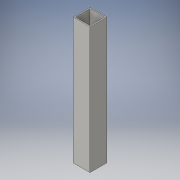
# Autodesk Inventor part: gripper arm bracket
Saved by Autodesk Inventor 2016 SP2 (Build 200236200, 236)
## iProperties
Created: 2018-02-13
Part Number: gripper arm bracket
Material: Generic
Document SubType Name: Modeling
Designer: CAD
Density: 1 g/cm^3
Appearance: Default
Author: CAD
Autodesk Inventor part; units mm, degrees
ref_plane "YZ Plane" through (0, 0, 0) normal (1, 0, 0) x (0, 1, 0)
ref_plane "XZ Plane" through (0, 0, 0) normal (0, 1, 0) x (-1, 0, 0)
ref_plane "XY Plane" through (0, 0, 0) normal (0, 0, 1) x (1, 0, 0)
sketch "Sketch1" plane through (0, 0, 0) normal (0, 1, 0) x (-1, 0, 0)
  line L0 (12.7, 0) -> (12.7, -12.7)
  line L1 (12.7, -12.7) -> (0, -12.7)
  line L2 (0, 0) -> (24.2319, 0) construction
  line L3 (0, 0) -> (0, -21.2534) construction
  line L4 (12.7, 0) -> (12.7, 12.7)
  line L5 (12.7, 12.7) -> (0, 12.7)
  line L6 (-12.7, 0) -> (-12.7, -12.7)
  line L7 (-12.7, -12.7) -> (0, -12.7)
  line L8 (-12.7, 0) -> (-12.7, 12.7)
  line L9 (-12.7, 12.7) -> (0, 12.7)
  line L10 (0, -11.1125) -> (11.1125, -11.1125)
  line L11 (11.1125, -11.1125) -> (11.1125, 0)
  line L12 (11.1125, 0) -> (11.1125, 11.1125)
  line L13 (11.1125, 11.1125) -> (0, 11.1125)
  line L14 (0, 11.1125) -> (-11.1125, 11.1125)
  line L15 (-11.1125, 11.1125) -> (-11.1125, 0)
  line L16 (-11.1125, 0) -> (-11.1125, -11.1125)
  line L17 (-11.1125, -11.1125) -> (0, -11.1125)
  dimension "d1" = 12.7
  dimension "d2" = 12.7
  dimension "d3" = 12.7
  dimension "d4" = 12.7
  dimension "d5" = 24.2319
  dimension "d6" = 21.2534
  dimension "d7" = 1.5875
  constraints: 36 end point, 5 symmetric about line, 2 horizontal, 2 vertical, 7 other
  measures "d1" distance of L0.end L1.end
  measures "d2" distance of L0.start L0.end
  measures "d3" distance of L2.start L0.start
  measures "d4" distance from line of L2 L1.end
  measures "d5" distance of L2.start L2.end
  measures "d6" distance of L2.start L3.end
  measures "d7" distance between parallel lines of L1 L10
extrude "Extrusion1" add sketch "Sketch1" along normal blind 190.5
equation "\"d3\" = d1"
body "Solid1"
